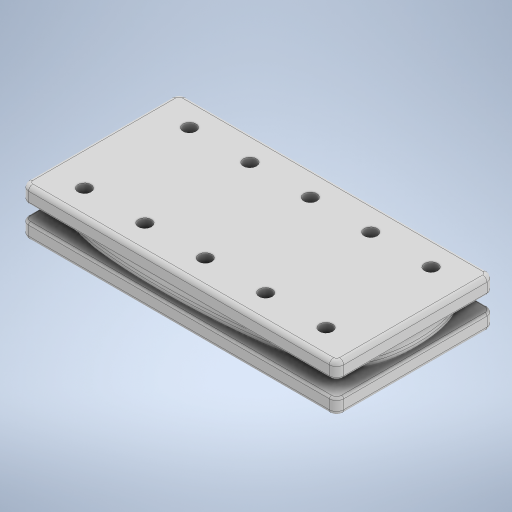
# Autodesk Inventor part: bourbon-biscuit-earings
Saved by Autodesk Inventor 2024.1 (Build 281209000, 209)
## iProperties
Created: 2025-02-21
Part Number: bourbon-biscuit-earings
Material: Generic
Document SubType Name: Modeling
Designer: iwheard
Density: 1 g/cm^3
Appearance: Default
Author: iwheard
Autodesk Inventor part; units mm, degrees
ref_plane "YZ Plane" through (0, 0, 0) normal (1, 0, 0) x (0, 1, 0)
ref_plane "XZ Plane" through (0, 0, 0) normal (0, 1, 0) x (-1, 0, 0)
sketch "Sketch1" plane through (0, 0, 0) normal (0, 1, 0) x (-1, 0, 0)
  line L0 (-0.1997, -30) -> (-60, -30)
  line L1 (-60, -30) -> (-60, 0)
  line L2 (-60, 0) -> (0, 0)
  line L3 (-8.6098, -2.2261) -> (-11.8789, -1.4947) construction
  line L4 (-6.3055, -2.7417) -> (-8.6098, -2.2261) construction
  spline S0 degree 4 poles (-8.6098, -2.2261) (-11.8789, -1.4947) (-27.1029, 0.6776) (-49.5398, -1.7009) (-58.9021, -4.7604) (-60, -16.0819) (-58.9021, -26.3466) (-51.8193, -28.7204) (-28.8089, -30) (-4.8111, -28.2226) (-2.611, -25.2524) (-0.1997, -15) (-2.1497, -3.6715) (-6.3055, -2.7417) (-8.6098, -2.2261) knots 1 1 1 1 1 1.008137 1.947514 2 3 3.401421 4 5 5.500323 5.914583 5.976873 6 6 6 6 6
  line L5 (0, 0) -> (-60, 0)
  line L6 (-60, 0) -> (-60, -30)
  line L7 (-60, -30) -> (0, -30)
  line L8 (0, -30) -> (0, 0)
  line L9 (-2.1497, -3.6715) -> (-6.3055, -2.7417) construction
  line L10 (-11.8789, -1.4947) -> (-27.1029, 0.6776) construction
  line L11 (-0.1997, -15) -> (-2.1497, -3.6715) construction
  line L12 (-28.8089, -30) -> (-4.8111, -28.2226) construction
  line L13 (-4.8111, -28.2226) -> (-2.611, -25.2524) construction
  line L14 (-2.611, -25.2524) -> (-0.1997, -15) construction
  line L15 (-60, -16.0819) -> (-58.9021, -26.3466) construction
  line L16 (-58.9021, -26.3466) -> (-51.8193, -28.7204) construction
  line L17 (-51.8193, -28.7204) -> (-28.8089, -30) construction
  line L18 (-27.1029, 0.6776) -> (-49.5398, -1.7009) construction
  line L19 (-49.5398, -1.7009) -> (-58.9021, -4.7604) construction
  line L20 (-58.9021, -4.7604) -> (-60, -16.0819) construction
  dimension "d1" = 30
  dimension "d9" = 60
  constraints: 14 end point, 3 parallel, 3 point on line, 2 horizontal, 2 perpendicular, 1 coincident, 2 other
  measures "d1" distance between parallel lines of L2 L0
  measures "d9" distance between parallel lines of L1 L8
extrude "Extrusion1" add sketch "Sketch1" along normal blind 3 contours S0
fillet "Fillet1" radius 1.225 2 edges at (54.5017, 3, -27.37) (54.5017, 0, -27.37)
ref_plane "Work Plane1" through (0, 1.5, 0) normal (0, 1, 0) x (1, 0, 0)
sketch "Sketch5" plane through (0, 3, 0) normal (0, 1, 0) x (1, 0, 0)
  line L0 (0.1997, 30) -> (60, 30) projected
  line L1 (0, 30) -> (0, 0) projected
  line L2 (60, 0) -> (0, 0) projected
  line L3 (60, 30) -> (60, 0) projected
  line L4 (0.1997, 30) -> (0, 30)
  constraints: 2 end point, 1 horizontal
extrude "Extrusion5" add sketch "Sketch5" along normal blind 3 separate body
fillet "Fillet2" radius 1.36 4 edges at (60, 4.5, 0) (0, 4.5, 0) (60, 4.5, -30) (0, 4.5, -30)
fillet "Fillet3" radius 0.4 8 edges at (0.3983, 3, -29.6017) (0, 3, -15) (0.3983, 3, -0.3983) (30, 3, 0) (59.6017, 3, -0.3983) (60, 3, -15) (59.6017, 3, -29.6017) (30, 3, -30)
fillet "Fillet4" radius 0.8 8 edges at (0.3983, 6, -29.6017) (0, 6, -15) (0.3983, 6, -0.3983) (30, 6, 0) (59.6017, 6, -0.3983) (60, 6, -15) (59.6017, 6, -29.6017) (30, 6, -30)
sketch "Sketch6" plane through (0, 6, 0) normal (0, 1, 0) x (1, 0, 0)
  circle A0 centre (7, 25) radius 1.25
  circle A1 centre (18.5, 25) radius 1.25
  circle A2 centre (30, 25) radius 1.25
  circle A3 centre (41.5, 25) radius 1.25
  circle A4 centre (53, 25) radius 1.25
  circle A5 centre (7, 5) radius 1.25
  circle A6 centre (18.5, 5) radius 1.25
  circle A7 centre (30, 5) radius 1.25
  circle A8 centre (53, 5) radius 1.25
  circle A9 centre (41.5, 5) radius 1.25
  line L0 (1.36, 0) -> (58.64, 0) projected
  line L1 (58.64, 30) -> (1.36, 30) projected
  line L2 (0, 28.64) -> (0, 1.36) projected
  line L3 (60, 1.36) -> (60, 28.64) projected
  point P0 (0, 0)
  dimension "d18" = 5
  dimension "d19" = 5
  dimension "d20" = 7
  dimension "d21" = 7
  dimension "d22" = 11.5
  dimension "d23" = 11.5
  dimension "d24" = 11.5
  dimension "d25" = 11.5
  dimension "d26" = 2.5
  constraints: 10 centre point, 9 equal radius, 8 horizontal alignment, 5 vertical alignment
  measures "d18" distance from line of L0 A5.centre
  measures "d19" distance from line of L1 A0.centre
  measures "d20" distance from line of A0.centre L2
  measures "d21" distance from line of A4.centre L3
  measures "d22" distance of A4.centre A3.centre
  measures "d23" distance of A3.centre A2.centre
  measures "d24" distance of A1.centre A2.centre
  measures "d25" distance of A0.centre A1.centre
  measures "d26" diameter of A0
extrude "Extrusion6" cut sketch "Sketch6" against normal blind 3 bodies 2
mirror "Mirror1" about plane through (0, 1.5, 0) normal (0, 1, 0) of "Extrusion5", "Fillet3", "Extrusion6", "Fillet4", "Fillet2" bodies 1
equation "\"d21\" = d20"
equation "\"d23\" = d22"
equation "\"d24\" = d23"
body "Solid1"
